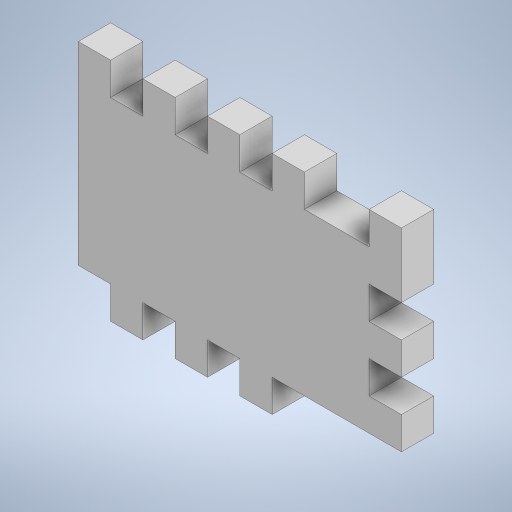
# Autodesk Inventor part: backside
Saved by Autodesk Inventor 2024 (Build 280153000, 153)
## iProperties
Created: 2024-04-15
Part Number: backside
Material: Generic
Document SubType Name: Modeling
Designer: srika
Density: 1 g/cm^3
Appearance: Default
Author: srika
Autodesk Inventor part; units mm, degrees
ref_plane "YZ Plane" through (0, 0, 0) normal (1, 0, 0) x (0, 1, 0)
ref_plane "XZ Plane" through (0, 0, 0) normal (0, 1, 0) x (-1, 0, 0)
ref_plane "XY Plane" through (0, 0, 0) normal (0, 0, 1) x (1, 0, 0)
sketch "Sketch2" plane through (0, 0, 0) normal (0, 0, 1) x (1, 0, 0)
  line L0 (5, 5) -> (10, 5)
  line L1 (10, 5) -> (10, 0)
  line L2 (10, 0) -> (5, 0)
  line L3 (5, 0) -> (5, 5)
  line L4 (0, 5) -> (40, 5)
  line L5 (40, 30) -> (0, 30)
  line L6 (0, 30) -> (0, 5)
  line L7 (20, 5) -> (20, 0)
  line L8 (20, 0) -> (15, 0)
  line L9 (15, 0) -> (15, 5)
  line L10 (30, 5) -> (30, 0)
  line L11 (30, 0) -> (25, 0)
  line L12 (25, 0) -> (25, 5)
  line L13 (10, 30) -> (5, 30)
  line L14 (20, 30) -> (15, 30)
  line L15 (30, 30) -> (25, 30)
  line L16 (0, 35) -> (5, 35)
  line L17 (5, 35) -> (5, 30)
  line L18 (5, 30) -> (0, 30)
  line L19 (0, 30) -> (0, 35)
  line L20 (15, 35) -> (15, 30)
  line L21 (15, 30) -> (10, 30)
  line L22 (10, 30) -> (10, 35)
  line L23 (10, 35) -> (15, 35)
  line L24 (25, 35) -> (25, 30)
  line L25 (25, 30) -> (20, 30)
  line L26 (20, 30) -> (20, 35)
  line L27 (20, 35) -> (25, 35)
  line L28 (35, 35) -> (35, 30)
  line L29 (35, 30) -> (30, 30)
  line L30 (30, 30) -> (30, 35)
  line L31 (30, 35) -> (35, 35)
  line L32 (40, 35) -> (50, 35)
  line L33 (50, 35) -> (50, 5)
  line L34 (50, 5) -> (40, 5)
  line L35 (40, 5) -> (40, 35)
  line L36 (40, 35) -> (45, 35)
  line L37 (45, 35) -> (45, 30)
  line L38 (45, 30) -> (40, 30)
  line L39 (40, 30) -> (40, 35)
  line L40 (45, 30) -> (50, 30)
  line L41 (50, 30) -> (50, 25)
  line L42 (50, 25) -> (45, 25)
  line L43 (45, 25) -> (45, 30)
  line L44 (40, 25) -> (45, 25)
  line L45 (45, 25) -> (45, 20)
  line L46 (45, 20) -> (40, 20)
  line L47 (40, 20) -> (40, 25)
  line L48 (45, 20) -> (50, 20)
  line L49 (50, 20) -> (50, 15)
  line L50 (50, 15) -> (45, 15)
  line L51 (45, 15) -> (45, 20)
  line L52 (40, 15) -> (45, 15)
  line L53 (45, 15) -> (45, 10)
  line L54 (45, 10) -> (40, 10)
  line L55 (40, 10) -> (40, 15)
  line L56 (45, 10) -> (50, 10)
  line L57 (50, 10) -> (50, 5)
  line L58 (50, 5) -> (45, 5)
  line L59 (45, 5) -> (45, 10)
  point P0 (0, 0)
  dimension "d105" = 10
  dimension "d115" = 10
  constraints: 120 end point, 19 parallel, 12 horizontal, 9 perpendicular, 4 point on line, 1 midpoint, 41 other
  measures "d105" distance of L1.end L7.end
  measures "d115" distance of L5.end point (10, 30)
extrude "Extrusion3" add sketch "Sketch2" along normal blind 5 contours L4 L6 L5 L35 L0 | L0 L1 L2 L3 | L4 L7 L8 L9 | L19 L16 L17 L5 | L4 L10 L11 L12 | L22 L23 L20 L5 | L35 L54 L59 L34 | L26 L27 L24 L5 | L59 L56 L33 L34 | L35 L52 L53 L54 | L35 L46 L51 L52 | L30 L31 L28 L5 | L51 L48 L33 L50 | L35 L44 L45 L46 | L35 L38 L43 L44 | L43 L40 L33 L42 | L37 L32 L33 L40
body "Solid3"
